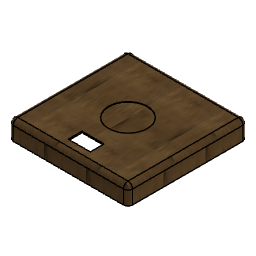
ESPressoScale (Autodesk Fusion 360 design; units mm, degrees)
Autodesk Fusion 360 part; units mm, degrees
note: some values were not read from the file. Set by a fixed rule: which face or edge a step refers to.
sketch "Skizze1" plane through (0, 0, 0) normal (0, 0, 1) x (1, 0, 0)
  line L0 (-22.5, 5) -> (22.5, 5)
  line L1 (22.5, 5) -> (22.5, -5)
  line L2 (22.5, -5) -> (-22.5, -5)
  line L3 (-22.5, -5) -> (-22.5, 5)
  circle A0 centre (-18.5, 0) radius 1.5
  circle A1 centre (-11.5, 0) radius 1.5
  circle A2 centre (18.5, 0) radius 1.5
  circle A3 centre (11.5, 0) radius 1.5
  dimension "d1" = 45
  dimension "d2" = 10
  dimension "d3" = 5
  dimension "d4" = 22.5
  dimension "d5" = 3
  dimension "d6" = 4
  dimension "d7" = 3
  dimension "d8" = 11
  dimension "d9" = 3
  dimension "d10" = 4
  dimension "d11" = 3
  dimension "d12" = 11
  constraint horizontal L0
  constraint vertical L1
  constraint horizontal L2
  constraint vertical L3
  measures "d1" distance of L0.start L0.end
  measures "d2" distance of L0.start L2.end
  measures "d3" distance of origin L0
  measures "d4" distance of origin L1
  measures "d5" diameter of A0
  measures "d6" distance of L3 A0.centre
  measures "d7" diameter of A1
  measures "d8" distance of L3 A1.centre
  measures "d9" diameter of A2
  measures "d10" distance of L1 A2.centre
  measures "d11" diameter of A3
  measures "d12" distance of L1 A3.centre
extrude "Extrusion1" add sketch "Skizze1" along normal blind 6 makes body 1
copy_body "Körper->Berechn1" bodies 1 removing the originals makes body 2 in component "300gWaegezelle"
sketch "Skizze2" plane through (0, 0, 0) normal (0, 0, 1) x (1, 0, 0)
  line L0 (-65, 65) -> (65, 65)
  line L1 (65, 65) -> (65, -65)
  line L2 (65, -65) -> (-65, -65)
  line L3 (-65, -65) -> (-65, 65)
  dimension "d15" = 130
  dimension "d16" = 130
  dimension "d17" = 65
  dimension "d18" = 65
  constraint horizontal L0
  constraint vertical L1
  constraint horizontal L2
  constraint vertical L3
  measures "d15" distance of L0.start L0.end
  measures "d16" distance of L0.start L2.end
  measures "d17" distance of origin L0
  measures "d18" distance of origin L3
ref_plane "Arbeitsebene1" through (0, 0, 25) normal (0, 0, 1) x (1, 0, 0)
extrude "Extrusion2" add sketch "Skizze2" against normal blind 20 from surface at 25 separate body makes body 3
fillet "Abrundung1" radius 5 8 edges at (-65, 0, 25) (0, 65, 25) (65, 0, 25) (0, -65, 25) (65, -65, 15) (-65, -65, 15) (-65, 65, 15) (65, 65, 15) on bodies 3
shell "Schale1" thickness 3 removed faces 1 at (-23.3333, -21.6667, 5) on bodies 3
extrude "Extrusion3" add 1 faces at (-20, 20, 22) along direction (0, 0, 1) blind 18 from surface at -22 on bodies 3 bodies 3 makes body 4
fillet "Abrundung2" radius 5 4 edges at (60, 60, 9) (-60, 60, 9) (-60, -60, 9) (60, -60, 9) on bodies 4
shell "Schale2" thickness 1.6 outward thickness 0.2 removed faces 1 at (18.3333, -20, 18) on bodies 4
move_body "Verschieben1" bodies 2 to x (1, 0, 0) y (0, 1, 0) z (0, 0, 1) at (0, 0, 8) in component "300gWaegezelle"
sketch "Skizze3" plane through (0, 0, 25) normal (0, 0, 1) x (-1, 0, 0)
  line L0 (60, 60) -> (-60, 60)
  line L1 (-60, 60) -> (-60, -60)
  line L2 (-60, -60) -> (60, -60)
  line L3 (60, -60) -> (60, 60)
  line L4 (24.5, -7) -> (8.5, -7)
  line L5 (8.5, -7) -> (8.5, 7)
  line L6 (8.5, 7) -> (24.5, 7)
  line L7 (24.5, 7) -> (24.5, -7)
  circle A0 centre (0, 0) radius 21
  circle A1 centre (11.5, 0) radius 2.3
  circle A2 centre (18.5, 0) radius 2.3
  line L8 (45, 35) -> (31, 35)
  line L9 (31, 35) -> (31, 53)
  line L10 (31, 53) -> (45, 53)
  line L11 (45, 53) -> (45, 35)
  line L12 (-45, 35) -> (-31, 35)
  line L13 (-31, 35) -> (-31, 53)
  line L14 (-31, 53) -> (-45, 53)
  line L15 (-45, 53) -> (-45, 35)
  line L16 (12, 38) -> (-12, 38)
  line L17 (-12, 38) -> (-12, 53)
  line L18 (-12, 53) -> (12, 53)
  line L19 (12, 53) -> (12, 38)
  line L20 (12, 53) -> (-15, 53)
  line L21 (20, 33) -> (-20, 33)
  line L22 (-20, 33) -> (-20, 29)
  line L23 (-20, 29) -> (20, 29)
  line L24 (20, 29) -> (20, 33)
  dimension "d33" = 42
  dimension "d39" = 14
  dimension "d40" = 18
  dimension "d41" = 15
  dimension "d42" = 95
  dimension "d43" = 14
  dimension "d44" = 18
  dimension "d45" = 95
  dimension "d46" = 15
  dimension "d47" = 24
  dimension "d48" = 15
  dimension "d49" = 12
  dimension "d50" = 98
  dimension "d91" = 4.6
  dimension "d92" = 4.6
  dimension "d93" = 7
  dimension "d94" = 7
  dimension "d111" = 40
  dimension "d112" = 4
  dimension "d113" = 20
  dimension "d114" = 20
  constraint horizontal L4
  constraint vertical L5
  constraint horizontal L6
  constraint vertical L7
  constraint coincident A0.centre origin
  constraint horizontal L8
  constraint vertical L9
  constraint horizontal L10
  constraint vertical L11
  constraint horizontal L12
  constraint vertical L13
  constraint horizontal L14
  constraint vertical L15
  constraint horizontal L16
  constraint vertical L17
  constraint horizontal L18
  constraint vertical L19
  constraint horizontal L20
  constraint horizontal L21
  constraint vertical L22
  constraint horizontal L23
  constraint vertical L24
  measures "d33" diameter of A0
  measures "d39" distance of L8.start L8.end
  measures "d40" distance of L8.start L10.end
  measures "d41" distance of L3 L11
  measures "d42" distance of L2 L8
  measures "d43" distance of L12.start L12.end
  measures "d44" distance of L12.start L14.end
  measures "d45" distance of L2 L12
  measures "d46" distance of L1 L15
  measures "d47" distance of L16.start L16.end
  measures "d48" distance of L16.start L18.end
  measures "d49" distance of A0.centre L19
  measures "d50" distance of L2 L16
  measures "d91" diameter of A2
  measures "d92" diameter of A1
  measures "d93" distance of L0 L18
  measures "d94" distance of L0 L10
  measures "d111" distance of L21.start L21.end
  measures "d112" distance of L21.start L23.end
  measures "d113" distance of A0.centre L22
  measures "d114" distance of L20 L21
extrude "Extrusion4" add sketch "Skizze3" along normal up to surface (8 mm away) from surface at -11 contours L4 L6 L7 A0 | L4 L5 L6 A0 picked at (13.5464, 5.3803) bodies 3
extrude "Extrusion5" cut sketch "Skizze3" against normal blind 0.5 contours L4 L5 L6 A0 | L4 L5 L6 A0 | A1 | A2 bodies 3
extrude "Extrusion6" cut sketch "Skizze3" against normal blind 10 contours L16 L17 L18 L19 L20 bodies 3
extrude "Extrusion7" cut sketch "Skizze3" along normal blind 1.8 from surface at -3 contours L8 L9 L10 L11 | L12 L13 L14 L15 bodies 3
sketch "Skizze4" plane through (0, 0, 1.6) normal (0, 0, 1) x (-1, 0, 0)
  arc A0 (-55, 58.4) -> (-58.4, 55) centre (-55, 55) ccw
  line L0 (-58.4, 55) -> (-58.4, -55)
  arc A1 (-58.4, -55) -> (-55, -58.4) centre (-55, -55) ccw
  line L1 (-55, -58.4) -> (55, -58.4)
  arc A2 (55, -58.4) -> (58.4, -55) centre (55, -55) ccw
  line L2 (58.4, -55) -> (58.4, 55)
  arc A3 (58.4, 55) -> (55, 58.4) centre (55, 55) ccw
  line L3 (55, 58.4) -> (-55, 58.4)
  line L4 (-22.5, 5) -> (-9, 5)
  line L5 (-9, 5) -> (-9, -5)
  line L6 (-9, -5) -> (-22.5, -5)
  line L7 (-22.5, -5) -> (-22.5, 5)
  circle A4 centre (-18.5026, 0.0003) radius 1.75
  circle A5 centre (-11.4986, -0.0024) radius 1.75
  circle A6 centre (-32.5, -53.4) radius 1
  circle A7 centre (-32.5, -53.4) radius 3
  circle A8 centre (32.5, -53.4) radius 1
  circle A9 centre (32.5, -53.4) radius 3
  circle A10 centre (-32.5, -27.4) radius 1
  circle A11 centre (-32.5, -27.4) radius 3
  circle A12 centre (32.5, -27.4) radius 1
  circle A13 centre (32.5, -27.4) radius 3
  line L8 (-50.4, 11.6) -> (-35.4, 11.6)
  line L9 (-35.4, 11.6) -> (-35.4, -3.4)
  line L10 (-35.4, -3.4) -> (-50.4, -3.4)
  line L11 (-50.4, -3.4) -> (-50.4, 11.6)
  line L12 (-52.4, 13.6) -> (-33.4, 13.6)
  line L13 (-33.4, 13.6) -> (-33.4, -5.4)
  line L14 (-33.4, -5.4) -> (-52.4, -5.4)
  line L15 (-52.4, -5.4) -> (-52.4, 13.6)
  line L16 (57.4, 3) -> (37.4, 3)
  line L17 (37.4, 3) -> (37.4, -3)
  line L18 (37.4, -3) -> (57.4, -3)
  line L19 (57.4, -3) -> (57.4, 3)
  line L20 (51.4, 3) -> (45.4, 3)
  line L21 (45.4, 3) -> (45.4, -3)
  line L22 (45.4, -3) -> (51.4, -3)
  line L23 (51.4, -3) -> (51.4, 3)
  circle A14 centre (-18.5026, 0.0003) radius 3.25
  circle A15 centre (-11.4986, -0.0024) radius 3.25
  dimension "d56" = 3.5
  dimension "d57" = 3.5
  dimension "d58" = 2
  dimension "d59" = 32.5
  dimension "d60" = 6
  dimension "d63" = 65
  dimension "d64" = 26
  dimension "d72" = 15
  dimension "d73" = 15
  dimension "d74" = 8
  dimension "d75" = 55
  dimension "d76" = 93.8
  dimension "d77" = -2
  dimension "d80" = 5
  dimension "d81" = 20
  dimension "d82" = 6
  dimension "d83" = 3
  dimension "d84" = 1
  dimension "d85" = 6
  dimension "d86" = 6
  dimension "d118" = 6.5
  dimension "d119" = 6.5
  constraint horizontal L4
  constraint vertical L5
  constraint horizontal L6
  constraint vertical L7
  constraint concentric A6 A7
  constraint horizontal L8
  constraint vertical L9
  constraint horizontal L10
  constraint vertical L11
  constraint horizontal L16
  constraint vertical L17
  constraint horizontal L18
  constraint vertical L19
  constraint horizontal L20
  constraint vertical L21
  constraint horizontal L22
  constraint vertical L23
  constraint coincident L16 L20.start
  constraint concentric A4 A14
  constraint concentric A5 A15
  measures "d56" diameter of A4
  measures "d57" diameter of A5
  measures "d58" diameter of A6
  measures "d59" horizontal distance of origin A6.centre
  measures "d60" diameter of A7
  measures "d72" distance of L8.start L8.end
  measures "d73" distance of L8.start L10.end
  measures "d74" distance of L0 L11
  measures "d75" distance of L1 L10
  measures "d76" distance of L2 L9
  measures "d80" distance of L1 A6.centre
  measures "d81" distance of L16.start L16.end
  measures "d82" distance of L16.start L18.end
  measures "d83" distance of origin L16
  measures "d84" distance of L2 L19
  measures "d85" distance of L20.start L20.end
  measures "d86" distance of L19 L23
  measures "d118" diameter of A14
  measures "d119" diameter of A15
extrude "Extrusion1'" add sketch "Skizze4" along normal up to surface (6.4 mm away) separate body contours L4 L5 L6 L7 A15 | L5 A15 | A14 picked at (-9.2495, -0.0024) makes body 5 in component "300gWaegezelle"
combine "Kombinieren1" operation add target body 4 tool bodies 5
move_face "Flächen versetzen1" offset 2 1 faces at (13.5, 5, 3.7333) on bodies 4
move_face "Flächen versetzen2" offset 2 1 faces at (22.5, 3, 3.7333) on bodies 4
move_face "Flächen versetzen3" offset 2 1 faces at (14.1667, -5, 5.8667) on bodies 4
extrude "Extrusion8" add sketch "Skizze4" along normal blind 6 contours A7 | A9 | A11 | A13 bodies 4
extrude "Extrusion9" add sketch "Skizze4" along normal blind 4 contours L8 L9 L10 L11 bodies 4
extrude "Extrusion10" add sketch "Skizze4" along normal blind 15 contours L16 L18 L19 L23 | L16 L17 L18 L21 bodies 4
extrude "Extrusion11" add sketch "Skizze4" along normal blind 10 contours L16 L18 L20 L21 L22 L23 bodies 4
sketch "Skizze5" plane through (0, 0, 22) normal (0, 0, -1) x (1, 0, 0)
  line L0 (60, 60) -> (-60, 60)
  line L1 (-60, 60) -> (-60, -60)
  line L2 (-60, -60) -> (60, -60)
  line L3 (60, -60) -> (60, 60)
  line L4 (-8.5, 7) -> (-8.5, -7)
  line L5 (-8.5, -7) -> (-24.5, -7)
  line L6 (-24.5, -7) -> (-24.5, 7)
  line L7 (-24.5, 7) -> (-8.5, 7)
  line L8 (12, 53) -> (12, 38)
  line L9 (12, 38) -> (-12, 38)
  line L10 (-12, 38) -> (-12, 53)
  line L11 (-45, 53) -> (-31, 53)
  line L12 (-31, 53) -> (-31, 35)
  line L13 (-31, 35) -> (-45, 35)
  line L14 (-45, 35) -> (-45, 53)
  line L15 (45, 53) -> (45, 35)
  line L16 (45, 35) -> (31, 35)
  line L17 (31, 35) -> (31, 53)
  line L18 (31, 53) -> (45, 53)
  line L19 (-17.5, 55) -> (17.5, 55)
  line L20 (17.5, 55) -> (17.5, 35)
  line L21 (17.5, 35) -> (-17.5, 35)
  line L22 (-17.5, 35) -> (-17.5, 55)
  line L23 (-12, 53) -> (12, 53)
  line L24 (-17.5, 55) -> (17.5, 55)
  line L25 (17.5, 55) -> (17.5, 63)
  line L26 (17.5, 63) -> (-17.5, 63)
  line L27 (-17.5, 63) -> (-17.5, 55)
  dimension "d102" = 35
  dimension "d103" = 20
  dimension "d104" = 17.5
  dimension "d105" = 5
  dimension "d125" = 8
  constraint horizontal L19
  constraint vertical L20
  constraint horizontal L21
  constraint vertical L22
  constraint horizontal L24
  constraint vertical L25
  constraint horizontal L26
  constraint vertical L27
  measures "d102" distance of L19.start L19.end
  measures "d103" distance of L19.start L21.end
  measures "d104" distance of origin L20
  measures "d105" distance of L0 L19
  measures "d125" distance of L19.start L26.end
extrude "Extrusion13" cut sketch "Skizze5" against normal blind 1.5 contours L19 L20 L21 L22 L24 bodies 3
extrude "Extrusion14" add sketch "Skizze3" against normal blind 1.5 from surface at -3 contours L21 L22 L23 L24 bodies 3
chamfer "Fase1" distance 6 angle 45 1 edges at (9, 0, 1.6) on bodies 4
extrude "Extrusion15" cut sketch "Skizze4" along normal blind 5 from surface at -1.8 contours L5 A15 | L5 A15 | A4 | A5 | A14 bodies 4
chamfer "Fase2" distance 8 angle 45 1 edges at (-8.5, 0, 22) on bodies 3
extrude "Extrusion16" add sketch "Skizze5" along normal blind 1.5 contours L0 L19 L24 L25 L27 | L0 L25 L26 L27 bodies 3
extrude "Extrusion17" add sketch "Skizze5" against normal blind 0.7 separate body contours L19 L20 L21 L22 L24 makes body 6
extrude "Extrusion18" add sketch "Skizze5" against normal blind 2 contours L8 L9 L10 L23 bodies 6
extrude "Extrusion19" cut 1 faces at (-37.4, -1, 11.6) along direction (-1, 0, 0) blind 2 on bodies 4 bodies 4
chamfer "Fase3" distance 2 distance2 3 3 edges at (-29.703, 52.3152, 1.6) (-29.703, 26.3152, 1.6) (35.297, 52.3152, 1.6) measured on face at (1, -41.2667, 1.6) measured on face at (1, -41.2667, 1.6) measured on face at (1, -41.2667, 1.6) on bodies 4
extrude "Extrusion20" add 1 faces at (-57.4, 1, 11.6) along direction (-1, 0, 0) up to surface (1 mm away) on bodies 4 bodies 4
sketch "Skizze7" plane through (0, 0, 1.6) normal (0, 0, 1) x (-1, 0, 0)
  line L0 (-3, -7) -> (-24.5, -7)
  line L1 (-24.5, -7) -> (-24.5, 7)
  line L2 (-24.5, 7) -> (-3, 7)
  line L3 (-3, 7) -> (-3, -7)
  line L4 (-50.4, -3.4) -> (-50.4, 11.6)
  line L5 (-50.4, 11.6) -> (-35.4, 11.6)
  line L6 (-35.4, 11.6) -> (-35.4, -3.4)
  line L7 (-35.4, -3.4) -> (-50.4, -3.4)
  line L8 (39.4, 3) -> (58.4, 3)
  line L9 (58.4, 3) -> (58.4, 55)
  arc A0 (58.4, 55) -> (55, 58.4) centre (55, 55) ccw
  line L10 (55, 58.4) -> (-55, 58.4)
  arc A1 (-55, 58.4) -> (-58.4, 55) centre (-55, 55) ccw
  line L11 (-58.4, 55) -> (-58.4, -55)
  arc A2 (-58.4, -55) -> (-55, -58.4) centre (-55, -55) ccw
  line L12 (-55, -58.4) -> (-32.5, -58.4)
  circle A3 centre (-32.5, -53.4) radius 5
  line L13 (-32.5, -58.4) -> (32.5, -58.4)
  circle A4 centre (32.5, -53.4) radius 5
  line L14 (32.5, -58.4) -> (55, -58.4)
  arc A5 (55, -58.4) -> (58.4, -55) centre (55, -55) ccw
  line L15 (58.4, -55) -> (58.4, -3)
  line L16 (58.4, -3) -> (39.4, -3)
  line L17 (39.4, -3) -> (39.4, 3)
  circle A6 centre (-32.5, -27.4) radius 3
  circle A7 centre (32.5, -27.4) radius 5
  line L18 (23, -54.7754) -> (-23, -54.7754)
  line L19 (-25, -52.7754) -> (-25, -26.7754)
  line L20 (-23, -24.7754) -> (23, -24.7754)
  line L21 (25, -26.7754) -> (25, -52.7754)
  line L22 (-18, 45) -> (18, 45)
  line L23 (20, 43) -> (20, 17)
  line L24 (18, 15) -> (-18, 15)
  line L25 (-20, 17) -> (-20, 43)
  arc A8 (18, 15) -> (20, 17) centre (18, 17) ccw
  arc A9 (-20, 17) -> (-18, 15) centre (-18, 17) ccw
  arc A10 (-18, 45) -> (-20, 43) centre (-18, 43) ccw
  arc A11 (20, 43) -> (18, 45) centre (18, 43) ccw
  line L26 (18, 16) -> (-18, 16)
  arc A12 (-19, 17) -> (-18, 16) centre (-18, 17) ccw
  line L27 (-19, 17) -> (-19, 43)
  arc A13 (-18, 44) -> (-19, 43) centre (-18, 43) ccw
  line L28 (-18, 44) -> (18, 44)
  arc A14 (19, 43) -> (18, 44) centre (18, 43) ccw
  line L29 (19, 43) -> (19, 17)
  arc A15 (18, 16) -> (19, 17) centre (18, 17) ccw
  arc A16 (-21.5, 17) -> (-18, 13.5) centre (-18, 17) ccw
  line L30 (18, 13.5) -> (-18, 13.5)
  arc A17 (18, 13.5) -> (21.5, 17) centre (18, 17) ccw
  line L31 (21.5, 43) -> (21.5, 17)
  arc A18 (21.5, 43) -> (18, 46.5) centre (18, 43) ccw
  line L32 (-18, 46.5) -> (18, 46.5)
  arc A19 (-18, 46.5) -> (-21.5, 43) centre (-18, 43) ccw
  line L33 (-21.5, 17) -> (-21.5, 43)
  arc A20 (23, -54.7754) -> (25, -52.7754) centre (23, -52.7754) ccw
  arc A21 (-25, -52.7754) -> (-23, -54.7754) centre (-23, -52.7754) ccw
  arc A22 (-23, -24.7754) -> (-25, -26.7754) centre (-23, -26.7754) ccw
  arc A23 (25, -26.7754) -> (23, -24.7754) centre (23, -26.7754) ccw
  point P0 (25, -54.7754)
  point P1 (25, -24.7754)
  point P2 (-20, 45)
  point P3 (20, 45)
  point P4 (-20, 15)
  dimension "d140" = 30
  dimension "d141" = 50
  dimension "d142" = 25
  dimension "d143" = 40
  dimension "d144" = 30
  dimension "d145" = 20
  dimension "d146" = 1
  dimension "d152" = 2
  dimension "d153" = 15
  dimension "d154" = 14.4
  dimension "d155" = 38.4
  dimension "d156" = -1.5
  dimension "d157" = 2
  constraint horizontal L18
  constraint vertical L19
  constraint horizontal L20
  constraint vertical L21
  constraint horizontal L22
  constraint vertical L23
  constraint horizontal L24
  constraint vertical L25
  constraint tangent L23 A8
  constraint tangent L24 A8
  constraint coincident P4 L24
  constraint coincident P4 L25
  constraint tangent L24 A9
  constraint tangent L25 A9
  constraint equal A8 A9
  constraint coincident P2 L22
  constraint coincident P2 L25
  constraint tangent L22 A10
  constraint tangent L25 A10
  constraint equal A8 A10
  constraint coincident P3 L22
  constraint coincident P3 L23
  constraint tangent L22 A11
  constraint tangent L23 A11
  constraint equal A8 A11
  constraint coincident P0 L18
  constraint coincident P0 L21
  constraint tangent L18 A20
  constraint tangent L21 A20
  constraint tangent L18 A21
  constraint tangent L19 A21
  constraint equal A20 A21
  constraint tangent L19 A22
  constraint tangent L20 A22
  constraint equal A20 A22
  constraint coincident P1 L20
  constraint coincident P1 L21
  constraint tangent L20 A23
  constraint tangent L21 A23
  constraint equal A20 A23
  measures "d140" distance of P0 P1
  measures "d141" distance of L19 L21
  measures "d142" horizontal distance of origin P0
  measures "d143" distance of P2 P3
  measures "d144" distance of P2 P4
  measures "d145" distance of origin L25
  measures "d152" radius of A8
  measures "d153" distance of origin L24
  measures "d154" distance of L10 L28
  measures "d155" distance of L11 L25
  measures "d157" radius of A20
extrude "Extrusion21" [suppressed]
extrude "Extrusion22" [suppressed]
extrude "Extrusion23" [suppressed]
component "300gWaegezelle" placed x (1, 0, 0) y (0, 1, 0) z (0, 0, 1) at (0, 0, 0)
hidden bodies 4 6
equation "d4 = ( 45 / 2 ) * 1 mm"
equation "d17 = ( 130 / 2 ) * 1 mm"
equation "d18 = ( 130 / 2 ) * 1 mm"
equation "d49 = ( 24 / 2 ) * 1 mm"
equation "d59 = ( 65 / 2 ) * 1 mm"
equation "d89 = 15 mm - 5 mm"
equation "d104 = ( 35 / 2 ) * 1 mm"
named bodies: "300gWaegezelle", "Top", "Bottom", "Glas"
